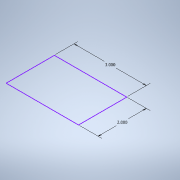
# Autodesk Inventor part: motor mount v2
Saved by Autodesk Inventor 2020 (Build 240168000, 168)
## iProperties
Created: 2021-02-27
Part Number: motor mount v2
Material: Generic
Document SubType Name: Modeling
Designer: Bernard Li
Density: 1 g/cm^3
Appearance: Default
Author: Bernard Li
Autodesk Inventor part; units mm, degrees
ref_plane "YZ Plane" through (0, 0, 0) normal (1, 0, 0) x (0, 1, 0)
ref_plane "XZ Plane" through (0, 0, 0) normal (0, 1, 0) x (-1, 0, 0)
ref_plane "XY Plane" through (0, 0, 0) normal (0, 0, 1) x (1, 0, 0)
sketch "Sketch3" plane through (0, 0, 0) normal (0, 1, 0) x (-1, 0, 0)
  line L0 (0.305195, 0) -> (-44.144805, 0)
  line L1 (-44.144805, 0) -> (-44.144805, -19.05)
  line L2 (-44.144805, -19.05) -> (0.305195, -19.05)
  line L3 (0.305195, -19.05) -> (0.305195, 0)
  arc A0 (-5.25, -6.73951) -> (-5.25, -5.26049) centre (-3.125, -6) ccw
  circle A1 centre (-3.125, -6) radius 2.25
  arc A2 (35.25, -5.26049) -> (35.25, -6.73951) centre (33.125, -6) ccw
  circle A3 centre (33.125, -6) radius 2.25
  line L4 (33.125, -6) -> (-3.125, -6)
  line L5 (0, -12) -> (0, 0)
  line L6 (30, -12) -> (0, -12)
  line L7 (0, -12) -> (0, 0)
  line L8 (0, 0) -> (30, 0)
  line L9 (30, 0) -> (30, -12)
  line L10 (30, -12) -> (0, 0) construction
  line L11 (0, -12) -> (30, 0) construction
  arc A4 (-42.475, -10.26451) -> (-42.475, -8.78549) centre (-40.35, -9.525) ccw
  circle A5 centre (-40.35, -9.525) radius 2.25
  arc A6 (-1.975, -8.78549) -> (-1.975, -10.26451) centre (-4.1, -9.525) ccw
  circle A7 centre (-4.1, -9.525) radius 2.25
  line L12 (-4.1, -9.525) -> (-40.35, -9.525)
  line L13 (-37.225, -15.525) -> (-37.225, -3.525)
  line L14 (-7.225, -15.525) -> (-37.225, -15.525)
  line L15 (-37.225, -15.525) -> (-37.225, -3.525)
  line L16 (-37.225, -3.525) -> (-7.225, -3.525)
  line L17 (-7.225, -3.525) -> (-7.225, -15.525)
  line L18 (-7.225, -15.525) -> (-37.225, -3.525) construction
  line L19 (-37.225, -15.525) -> (-7.225, -3.525) construction
  point P0 (15, -6)
  point P1 (-22.225, -9.525)
  point P2 (-4.875952, -7.413035)
  point P3 (-5.25, -6.73951)
  point P4 (-2.349048, -8.111965)
  point P5 (-1.975, -10.26451)
  point P6 (0.305195, -12)
  dimension "d12" = 4.5
  dimension "d13" = 4.5
  dimension "d17" = 4.5
  dimension "d18" = 4.5
  dimension "d9" = 44.45
  dimension "d10" = 19.05
  dimension "d11" = 36.25
  dimension "d14" = 30
  dimension "d15" = 12
  dimension "d16" = 36.25
  dimension "d19" = 30
  dimension "d20" = 12
  constraints: 40 end point, 8 point on circle, 6 midpoint, 6 parallel, 5 horizontal, 4 centre point, 4 coincident, 3 perpendicular, 12 other
  measures "d9" distance of L2.end L1.end
  measures "d10" distance of L1.end L0.end
  measures "d11" distance of L4.start L4.end
  measures "d14" distance of L5.end L8.end
  measures "d15" distance of L5.start L5.end
  measures "d16" distance of L12.start L12.end
  measures "d19" distance of L13.end L16.end
  measures "d20" distance of L13.start L13.end
extrude "Extrusion2" add sketch "Sketch3" along normal blind 3.81 contours L5 L6 L3 L2 L1 L0 | A0 A6 A1
sketch "Sketch4" plane through (0, 3.81, 0) normal (0, 1, 0) x (1, 0, 0)
  line L0 (0, 12) -> (0, 0)
  line L1 (-0.305195, 19.05) -> (-0.305195, 12)
  line L2 (0, 12) -> (-0.305195, 12)
  line L3 (-0.305195, 12) -> (-0.305195, 19.05)
  line L4 (-0.305195, 19.05) -> (0, 19.05)
  line L5 (0, 19.05) -> (0, 12)
  constraints: 8 end point, 2 parallel, 1 horizontal, 1 perpendicular
extrude "Extrusion3" cut sketch "Sketch4" against normal blind 3.81
sketch "Sketch5" plane through (0, 3.81, 0) normal (0, 1, 0) x (1, 0, 0)
  line L0 (44.144805, 19.05) -> (0, 19.05)
  line L1 (22.072403, 19.05) -> (22.072403, 0)
  line L2 (0, 0) -> (44.144805, 0)
  line L3 (22.072403, 9.525) -> (0, 9.525)
  line L4 (0, 19.05) -> (0, 0)
  circle A0 centre (3.999998, -4) radius 4
  circle A1 centre (3.999998, -4) radius 1.5
  line L5 (0, 0) -> (44.144805, 0)
  line L6 (0, -4.004242) -> (0, 0)
  line L7 (0, 0) -> (7.846401, 0)
  line L8 (7.846401, 0) -> (7.999998, -4.001295)
  circle A2 centre (3.999998, 23.05) radius 4
  circle A3 centre (3.999998, 23.05) radius 1.5
  line L9 (0, 23.054242) -> (0, 19.05)
  line L10 (0, 19.05) -> (7.846401, 19.05)
  line L11 (7.846401, 19.05) -> (7.999998, 23.051295)
  line L12 (44.144805, 19.05) -> (44.144805, 0)
  circle A4 centre (40.144808, -4) radius 4
  circle A5 centre (40.144808, -4) radius 1.5
  line L13 (44.144805, -4.004242) -> (44.144805, 0)
  line L14 (44.144805, 0) -> (36.298405, 0)
  line L15 (36.298405, 0) -> (36.144808, -4.001295)
  circle A6 centre (40.144808, 23.05) radius 4
  circle A7 centre (40.144808, 23.05) radius 1.5
  line L16 (44.144805, 23.054242) -> (44.144805, 19.05)
  line L17 (44.144805, 19.05) -> (36.298405, 19.05)
  line L18 (36.298405, 19.05) -> (36.144808, 23.051295)
  point P0 (44.144805, 9.525)
  point P1 (7.846401, 0)
  dimension "d25" = 8
  dimension "d26" = 3
  constraints: 30 end point, 23 symmetric about line, 8 centre point, 8 point on circle, 4 coincident, 4 midpoint, 2 point on line, 1 collinear, 1 equal length, 1 perpendicular, 1 tangent, 6 other
  measures "d25" diameter of A0
  measures "d26" diameter of A1
sketch "Sketch5 outline for Extrusion4" plane through (0, 3.81, 0) normal (0, 1, 0) x (1, 0, 0)
  line L0 (44.144805, -4.004242) -> (44.144805, 0)
  arc A0 (36.144808, -4.001295) -> (44.144805, -4.004242) centre (40.144808, -4) ccw
  line L1 (44.144805, 0) -> (36.298405, 0)
  line L2 (36.298405, 0) -> (36.144808, -4.001295)
  circle A1 centre (40.144808, -4) radius 1.5
  line L3 (36.298405, 19.05) -> (44.144805, 19.05)
  line L4 (36.144808, 23.051295) -> (36.298405, 19.05)
  line L5 (44.144805, 19.05) -> (44.144805, 23.054242)
  arc A2 (44.144805, 23.054242) -> (36.144808, 23.051295) centre (40.144808, 23.05) ccw
  circle A3 centre (40.144808, 23.05) radius 1.5
  line L6 (0, 0) -> (0, -4.004242)
  line L7 (7.846401, 0) -> (0, 0)
  arc A4 (0, -4.004242) -> (7.999998, -4.001295) centre (3.999998, -4) ccw
  line L8 (7.999998, -4.001295) -> (7.846401, 0)
  circle A5 centre (3.999998, -4) radius 1.5
  line L9 (7.846401, 19.05) -> (7.999998, 23.051295)
  line L10 (0, 19.05) -> (7.846401, 19.05)
  arc A6 (7.999998, 23.051295) -> (0, 23.054242) centre (3.999998, 23.05) ccw
  line L11 (0, 23.054242) -> (0, 19.05)
  circle A7 centre (3.999998, 23.05) radius 1.5
extrude "Extrusion4" add sketch "Sketch5 outline for Extrusion4" against normal blind 3.81
sketch "Sketch6" plane through (0, 3.81, 0) normal (0, 1, 0) x (1, 0, 0)
  line L0 (0, -7.9375) -> (44.144805, -7.9375)
  line L1 (44.144805, -7.9375) -> (44.144805, 26.9875)
  line L2 (44.144805, 26.9875) -> (0, 26.9875)
  line L3 (0, 26.9875) -> (0, -7.9375)
  circle A0 centre (3.999998, 23.05) radius 1.5
  circle A1 centre (3.999998, 23.05) radius 1.5
  circle A2 centre (3.999998, -4) radius 1.5
  circle A3 centre (3.999998, -4) radius 1.5
  circle A4 centre (40.144808, -4) radius 1.5
  circle A5 centre (40.144808, -4) radius 1.5
  circle A6 centre (40.144808, 23.05) radius 1.5
  circle A7 centre (40.144808, 23.05) radius 1.5
  constraints: 8 end point, 4 centre point, 4 coincident, 2 parallel, 1 horizontal, 1 perpendicular
body "Solid2"
